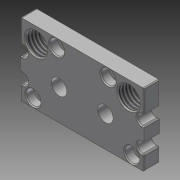
# Autodesk Inventor part: Rotary Pneumatic Cylinder Back End
Saved by Autodesk Inventor 2014 SP1 (Build 180222100, 222)
## iProperties
Created: 2013-12-16
Part Number: Rotary Pneumatic Cylinder Back End
Material: Generic
Document SubType Name: Modeling
Designer: Moses
Density: 1 g/cm^3
Appearance: Steel
Mass: 25.661 g
Surface Area: 101.918 cm^2
Volume: 25.661 cm^3
Author: Moses
Autodesk Inventor part; units mm, degrees
ref_plane "YZ Plane" through (0, 0, 0) normal (1, 0, 0) x (0, 1, 0)
ref_plane "XZ Plane" through (0, 0, 0) normal (0, 1, 0) x (-1, 0, 0)
ref_plane "XY Plane" through (0, 0, 0) normal (0, 0, 1) x (1, 0, 0)
sketch "Sketch1" plane through (0, 0, 0) normal (0, 0, 1) x (1, 0, 0)
  line L0 (0, 0) -> (0, 8.89)
  line L1 (0, 8.89) -> (1.27, 8.89)
  line L2 (1.27, 15.24) -> (0, 15.24)
  line L3 (0, 23.8125) -> (1.27, 23.8125)
  line L4 (1.27, 30.1625) -> (0, 30.1625)
  line L5 (0, 30.1625) -> (0, 44.45)
  line L6 (0, 44.45) -> (38.1, 44.45)
  line L7 (38.1, 44.45) -> (38.1, 0)
  line L8 (38.1, 0) -> (0, 0)
  arc A0 (1.27, 23.8125) -> (1.27, 30.1625) centre (1.27, 26.9875) ccw
  arc A1 (1.27, 8.89) -> (1.27, 15.24) centre (1.27, 12.065) ccw
  line L9 (0, 23.8125) -> (0, 15.24)
  circle A2 centre (7.62, 5.08) radius 4.445
  circle A3 centre (22.225, 39.37) radius 4.445
  circle A4 centre (9.525, 34.925) radius 6.731
  circle A5 centre (23.8125, 19.05) radius 4.7625
  circle A6 centre (22.225, 39.37) radius 2.3813
  circle A7 centre (7.62, 5.08) radius 2.3813
  dimension "d0" = 3.175
  dimension "d1" = 44.45
  dimension "d4" = 1.27
  dimension "d5" = 38.1
  dimension "d11" = 12.065
  dimension "d12" = 17.4625
  dimension "d13" = 8.89
  dimension "d14" = 7.62
  dimension "d15" = 5.08
  dimension "d18" = 22.225
  dimension "d19" = 5.08
  dimension "d20" = 13.462
  dimension "d21" = 9.525
  dimension "d22" = 19.05
  dimension "d23" = 9.525
  dimension "d24" = 9.525
  dimension "d25" = 4.7625
  constraints: 20 end point, 8 centre point, 5 horizontal, 4 point on circle, 4 tangent, 4 vertical, 3 equal radius, 3 parallel, 2 coincident, 1 perpendicular
  measures "d0" radius of A1
  measures "d1" distance between parallel lines of L8 L6
  measures "d4" distance of L0.end L1.end
  measures "d5" distance of L7.end L0.start
  measures "d11" distance from line of L8 A1.centre
  measures "d12" distance from line of L6 A0.centre
  measures "d13" diameter of A2
  measures "d14" distance from line of A2.centre L0
  measures "d15" distance from line of L8 A2.centre
  measures "d18" horizontal distance of L5.end A3.centre
  measures "d19" distance from line of L6 A3.centre
  measures "d20" diameter of A4
  measures "d21" diameter of A5
  measures "d22" distance from line of L8 A5.centre
  measures "d23" distance from line of A4.centre L5
  measures "d24" distance from line of A4.centre L6
  measures "d25" diameter of A6
extrude "Extrusion1" add sketch "Sketch1" against normal blind 9.525 contours L0 L1 A1 L2 L9 L3 A0 L4 L5 L6 L7 L8 | A2 | A3
extrude "Extrusion2" cut sketch "Sketch1" against normal blind 5.08 contours A2 | A3 | A6 | A7
fillet "Fillet1" radius 0.635 25 edges at (0, 15.24, -4.7625) (0, 23.8125, -4.7625) (0, 30.1625, -4.7625) (0, 8.89, -4.7625) (0, 0, -4.7625) (0, 44.45, -4.7625) (0, 37.3063, -9.525) (0.635, 23.8125, -9.525) (0.635, 30.1625, -9.525) (4.445, 26.9875, -9.525) (0.635, 8.89, -9.525) (0.635, 15.24, -9.525) (4.445, 12.065, -9.525) (0, 4.445, -9.525) (0, 37.3063, 0) (4.445, 26.9875, 0) (0.635, 23.8125, 0) (0.635, 30.1625, 0) (4.445, 12.065, 0) (0.635, 8.89, 0) (0.635, 15.24, 0) (0, 4.445, 0) (3.175, 5.08, 0) (17.78, 39.37, 0) (2.794, 34.925, 0)
thread "Thread1" size "10-32 UNF" class "2B" standard "ANSI Unified Screw Threads" full length
thread "Thread2" size "10-32 UNF" class "2B" standard "ANSI Unified Screw Threads" full length
thread "Thread3" size "9/16-12 UNC" class "2B" standard "ANSI Unified Screw Threads" full length
mirror "Mirror1" about plane through (38.1, 44.45, 0) normal (1, 0, 0)
body "Solid1"
